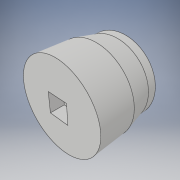
# Autodesk Inventor part: Power_Button
Saved by Autodesk Inventor 2019 (Build 230136000, 136)
## iProperties
Created: 2025-01-19
Part Number: Power_Button
Material: Générique
Document SubType Name: Modeling
Designer: Maxime
Density: 1 g/cm^3
Appearance: Par défaut
Author: Maxime
Autodesk Inventor part; units mm, degrees
ref_plane "YZ Plane" through (0, 0, 0) normal (1, 0, 0) x (0, 1, 0)
ref_plane "XZ Plane" through (0, 0, 0) normal (0, 1, 0) x (-1, 0, 0)
ref_plane "XY Plane" through (0, 0, 0) normal (0, 0, 1) x (1, 0, 0)
sketch "Esquisse1" plane through (0, 0, 0) normal (0, 0, 1) x (1, 0, 0)
  circle A0 centre (0, 0) radius 6.925
  dimension "d0" = 13.85
  constraints: 1 centre point, 1 coincident
  measures "d0" diameter of A0
extrude "Extrusion1" add sketch "Esquisse1" along normal blind 10.15 draft 10
sketch "Esquisse2" plane through (0, 0, 10.15) normal (0, 0, 1) x (1, 0, 0)
  line L0 (1.8, -1.8) -> (-1.8, -1.8)
  line L1 (-1.8, -1.8) -> (-1.8, 1.8)
  line L2 (-1.8, 1.8) -> (1.8, 1.8)
  line L3 (1.8, 1.8) -> (1.8, -1.8)
  line L4 (1.8, -1.8) -> (-1.8, 1.8) construction
  line L5 (-1.8, -1.8) -> (1.8, 1.8) construction
  point P0 (0, 0)
  dimension "d3" = 3.6
  dimension "d4" = 3.6
  constraints: 12 end point, 2 midpoint, 2 parallel, 1 horizontal, 1 perpendicular
  measures "d3" distance of L1.end L2.end
  measures "d4" distance of L0.end L1.end
extrude "Extrusion2" cut sketch "Esquisse2" against normal blind 2.5
ref_plane "Plan de construction1" through (0, 0, 4) normal (0, 0, -1) x (-1, 0, 0)
sketch "Esquisse3" plane through (0, 0, 4) normal (0, 0, -1) x (-1, 0, 0)
  circle A0 centre (0, 0) radius 7.6303 projected
  circle A1 centre (0, 0) radius 13.8909
  constraints: 1 centre point, 1 coincident
extrude "Extrusion3" cut sketch "Esquisse3" against normal through all
sketch "Esquisse4" plane through (0, 0, 0) normal (0, 0, -1) x (-1, 0, 0)
  circle A0 centre (0, 0) radius 6.925 projected
extrude "Extrusion4" add sketch "Esquisse4" along normal blind 1.6
sketch "Esquisse5" plane through (0, 0, -1.6) normal (0, 0, -1) x (-1, 0, 0)
  line L0 (2.6892, 4.9729) -> (2.6892, -4.9729) construction
  line L1 (2.6892, -4.9729) -> (-2.6892, -4.9729) construction
  line L2 (-2.6892, -4.9729) -> (-2.6892, 4.9729) construction
  line L3 (-2.6892, 4.9729) -> (2.6892, 4.9729) construction
  line L4 (10.6824, 0) -> (-10.6824, 0) projected
  line L5 (0, -10.6824) -> (0, 10.6824) projected
  spline S0 degree 2 poles (3.0556, 2.3545) (2.8465, 2.3545) (2.4673, 2.4882) (2.3409, 2.6122) knots 0 0 0 1 2 2 2
  spline S1 degree 2 poles (2.3409, 2.6122) (2.2606, 2.6876) (2.1294, 2.8724) (2.0832, 2.9818) knots 0 0 0 1 2 2 2
  spline S2 degree 2 poles (2.0832, 2.9818) (2.037, 3.0936) (1.9835, 3.3537) (1.9835, 3.5142) knots 0 0 0 1 2 2 2
  line L6 (1.9835, 3.5142) -> (1.9835, 3.908)
  line L7 (1.9835, 3.908) -> (1.0013, 3.908)
  line L8 (1.0013, 3.908) -> (1.0013, 4.6617)
  line L9 (1.0013, 4.6617) -> (4.0013, 4.6617)
  line L10 (4.0013, 4.6617) -> (4.0013, 3.4972)
  spline S3 degree 2 poles (4.0013, 3.4972) (4.0013, 3.2395) (3.9065, 2.8626) (3.8044, 2.7095) knots 0 0 0 1 2 2 2
  spline S4 degree 2 poles (3.8044, 2.7095) (3.6901, 2.5393) (3.3157, 2.3545) (3.0556, 2.3545) knots 0 0 0 1 2 2 2
  spline S5 degree 2 poles (3.0362, 3.1276) (3.165, 3.1276) (3.3473, 3.2492) (3.3814, 3.3318) knots 0 0 0 1 2 2 2
  spline S6 degree 2 poles (3.3814, 3.3318) (3.4276, 3.4388) (3.4422, 3.6333) (3.4422, 3.8011) knots 0 0 0 1 2 2 2
  line L11 (3.4422, 3.8011) -> (3.4422, 3.908)
  line L12 (3.4422, 3.908) -> (2.5426, 3.908)
  line L13 (2.5426, 3.908) -> (2.5426, 3.8545)
  spline S7 degree 2 poles (2.5426, 3.8545) (2.5426, 3.75) (2.5475, 3.5604) (2.5597, 3.4899) knots 0 0 0 1 2 2 2
  spline S8 degree 2 poles (2.5597, 3.4899) (2.5694, 3.4291) (2.6277, 3.2954) (2.6642, 3.2589) knots 0 0 0 1 2 2 2
  spline S9 degree 2 poles (2.6642, 3.2589) (2.7371, 3.1811) (2.9, 3.1276) (3.0362, 3.1276) knots 0 0 0 1 2 2 2
  line L14 (4.0013, -1.9169) -> (1.0013, -1.1584)
  line L15 (1.0013, -1.1584) -> (1.0013, -0.3318)
  line L16 (1.0013, -0.3318) -> (2.8563, 0.1495)
  line L17 (2.8563, 0.1495) -> (1.0013, 0.6139)
  line L18 (1.0013, 0.6139) -> (1.0013, 1.4429)
  line L19 (1.0013, 1.4429) -> (4.0013, 2.2014)
  line L20 (4.0013, 2.2014) -> (4.0013, 1.4186)
  line L21 (4.0013, 1.4186) -> (1.9932, 1.0053)
  line L22 (1.9932, 1.0053) -> (4.0013, 0.5045)
  line L23 (4.0013, 0.5045) -> (4.0013, -0.2443)
  line L24 (4.0013, -0.2443) -> (1.9908, -0.7208)
  line L25 (1.9908, -0.7208) -> (4.0013, -1.1536)
  line L26 (4.0013, -1.1536) -> (4.0013, -1.9169)
  line L27 (1.0013, -5.0604) -> (1.0013, -4.1438)
  line L28 (1.0013, -4.1438) -> (2.1026, -3.31)
  line L29 (2.1026, -3.31) -> (2.1026, -3.0377)
  line L30 (2.1026, -3.0377) -> (1.0013, -3.0377)
  line L31 (1.0013, -3.0377) -> (1.0013, -2.2889)
  line L32 (1.0013, -2.2889) -> (4.0013, -2.2889)
  line L33 (4.0013, -2.2889) -> (4.0013, -3.4947)
  spline S10 degree 2 poles (4.0013, -3.4947) (4.0013, -3.7451) (3.9381, -4.1147) (3.8409, -4.2727) knots 0 0 0 1 2 2 2
  spline S11 degree 2 poles (3.8409, -4.2727) (3.7388, -4.4331) (3.4203, -4.6228) (3.1772, -4.6228) knots 0 0 0 1 2 2 2
  spline S12 degree 2 poles (3.1772, -4.6228) (2.8344, -4.6228) (2.4041, -4.3116) (2.2777, -4.0515) knots 0 0 0 1 2 2 2
  line L34 (2.2777, -4.0515) -> (1.0013, -5.0604)
  spline S13 degree 2 poles (3.0824, -3.8497) (3.1966, -3.8497) (3.3595, -3.7622) (3.4033, -3.6625) knots 0 0 0 1 2 2 2
  spline S14 degree 2 poles (3.4033, -3.6625) (3.4324, -3.592) (3.4495, -3.4194) (3.4495, -3.2905) knots 0 0 0 1 2 2 2
  line L35 (3.4495, -3.2905) -> (3.4495, -3.0377)
  line L36 (3.4495, -3.0377) -> (2.6423, -3.0377)
  line L37 (2.6423, -3.0377) -> (2.6423, -3.2541)
  spline S15 degree 2 poles (2.6423, -3.2541) (2.6423, -3.4096) (2.6812, -3.6309) (2.742, -3.7062) knots 0 0 0 1 2 2 2
  spline S16 degree 2 poles (2.742, -3.7062) (2.8003, -3.7792) (2.9559, -3.8497) (3.0824, -3.8497) knots 0 0 0 1 2 2 2
  spline S17 degree 2 poles (-2.4381, 0.1374) (-3.1674, 0.1374) (-4.0013, 0.9153) (-4.0013, 1.5912) knots 0 0 0 1 2 2 2
  spline S18 degree 2 poles (-4.0013, 1.5912) (-4.0013, 2.2694) (-3.1577, 3.0425) (-2.4381, 3.0425) knots 0 0 0 1 2 2 2
  spline S19 degree 2 poles (-2.4381, 3.0425) (-1.7161, 3.0425) (-0.8749, 2.2694) (-0.8749, 1.5912) knots 0 0 0 1 2 2 2
  spline S20 degree 2 poles (-0.8749, 1.5912) (-0.8749, 0.9153) (-1.7112, 0.1374) (-2.4381, 0.1374) knots 0 0 0 1 2 2 2
  spline S21 degree 2 poles (-2.4381, 0.9153) (-2.1683, 0.9153) (-1.7914, 1.0247) (-1.6723, 1.1195) knots 0 0 0 1 2 2 2
  spline S22 degree 2 poles (-1.6723, 1.1195) (-1.5483, 1.2143) (-1.4413, 1.4575) (-1.4413, 1.5887) knots 0 0 0 1 2 2 2
  spline S23 degree 2 poles (-1.4413, 1.5887) (-1.4413, 1.7273) (-1.541, 1.9534) (-1.6674, 2.0579) knots 0 0 0 1 2 2 2
  spline S24 degree 2 poles (-1.6674, 2.0579) (-1.7841, 2.1503) (-2.1707, 2.2646) (-2.4381, 2.2646) knots 0 0 0 1 2 2 2
  spline S25 degree 2 poles (-2.4381, 2.2646) (-2.7153, 2.2646) (-3.0799, 2.1552) (-3.2039, 2.0604) knots 0 0 0 1 2 2 2
  spline S26 degree 2 poles (-3.2039, 2.0604) (-3.3279, 1.9656) (-3.4349, 1.72) (-3.4349, 1.5887) knots 0 0 0 1 2 2 2
  spline S27 degree 2 poles (-3.4349, 1.5887) (-3.4349, 1.455) (-3.3206, 1.2071) (-3.199, 1.1171) knots 0 0 0 1 2 2 2
  spline S28 degree 2 poles (-3.199, 1.1171) (-3.0678, 1.0199) (-2.7201, 0.9153) (-2.4381, 0.9153) knots 0 0 0 1 2 2 2
  line L38 (-3.9381, -2.8797) -> (-3.9381, -2.1552)
  line L39 (-3.9381, -2.1552) -> (-1.8473, -0.998)
  line L40 (-1.8473, -0.998) -> (-3.9381, -0.998)
  line L41 (-3.9381, -0.998) -> (-3.9381, -0.31)
  line L42 (-3.9381, -0.31) -> (-0.9381, -0.31)
  line L43 (-0.9381, -0.31) -> (-0.9381, -1.2338)
  line L44 (-0.9381, -1.2338) -> (-2.6569, -2.1917)
  line L45 (-2.6569, -2.1917) -> (-0.9381, -2.1917)
  line L46 (-0.9381, -2.1917) -> (-0.9381, -2.8797)
  line L47 (-0.9381, -2.8797) -> (-3.9381, -2.8797)
  point P0 (0, 0)
  point P1 (-3.9441, 0)
  point P2 (0, -4.9729)
  point P3 (-2.6892, 0)
  point P4 (0, -4.9729)
  constraints: 4 point on line, 2 midpoint, 2 other
extrude "Extrusion5" cut sketch "Esquisse5" against normal blind 0.15
